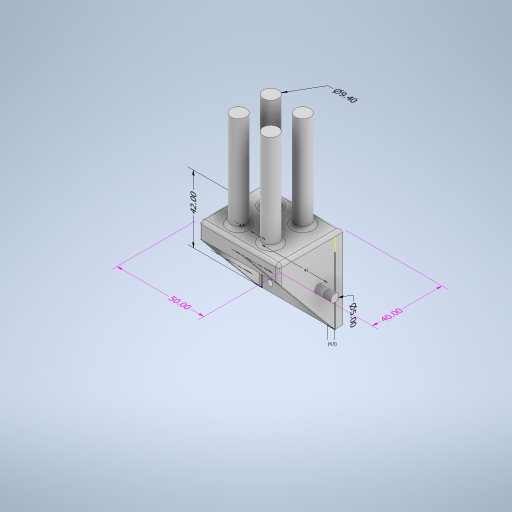
# Autodesk Inventor part: Attache moteur 3.0 renforcée
Saved by Autodesk Inventor 2023 (Build 270158000, 158)
## iProperties
Created: 2023-01-13
Part Number: Attache moteur 3.0 renforcée
Material: Générique
Document SubType Name: Modeling
Designer: pined
Density: 1 g/cm^3
Appearance: Par défaut
Mass: 44.8321 g
Surface Area: 196.652 cm^2
Volume: 44.8321 cm^3
Author: pined
Autodesk Inventor part; units mm, degrees
ref_plane "YZ Plane" through (0, 0, 0) normal (1, 0, 0) x (0, 1, 0)
ref_plane "XZ Plane" through (0, 0, 0) normal (0, 1, 0) x (-1, 0, 0)
ref_plane "XY Plane" through (0, 0, 0) normal (0, 0, 1) x (1, 0, 0)
sketch "Esquisse1" plane through (0, 0, 0) normal (1, 0, 0) x (0, 1, 0)
  line L0 (40.4154, 29.6476) -> (33.4154, 29.6476)
  line L1 (33.4154, 29.6476) -> (33.4154, -10.3524)
  line L2 (33.4154, -10.3524) -> (40.4154, -10.3524)
  line L3 (40.4154, -10.3524) -> (40.4154, 29.6476)
  line L4 (33.4154, -5.3524) -> (-16.5846, -5.3524)
  line L5 (-16.5846, -5.3524) -> (-16.5846, -10.3524)
  line L6 (-16.5846, -10.3524) -> (33.4154, -10.3524)
  line L7 (33.4154, -10.3524) -> (33.4154, -5.3524)
  point P0 (0, 0)
  point P1 (36.9154, -10.3524)
  point P2 (36.9154, 29.6476)
  point P3 (-16.5846, -7.8524)
  point P4 (33.4154, -7.8524)
  point P5 (33.4154, -10.3524)
  dimension "d0" = 40
  dimension "d1" = 7
  dimension "d2" = 5
  dimension "d3" = 50
  constraints: 16 end point, 4 midpoint, 4 parallel, 2 horizontal, 2 perpendicular, 1 point on line
  measures "d0" distance of point (36.915, -10.352) point (36.915, 29.648)
  measures "d1" distance between parallel lines of L1 L3
  measures "d2" distance between parallel lines of L6 L4
  measures "d3" distance of point (-16.585, -7.852) point (33.415, -7.852)
extrude "Extrusion1" add sketch "Esquisse1" along normal blind 50
sketch "Esquisse2" plane through (0, 33.4154, -5.3524) normal (0, -1, 0) x (1, 0, 0)
  line L0 (50, 35) -> (50, 0) projected
  line L1 (0, 0) -> (0, -5) projected
  line L2 (50, 35) -> (0, 0)
  line L3 (0, 0) -> (50, 0) projected
  line L4 (0, 35) -> (0, 0) projected
  line L5 (50, 0) -> (0, 35)
  line L6 (50, 3.0516) -> (4.3595, 35)
  line L7 (0, 35) -> (50, 35) projected
  line L8 (0, 31.9484) -> (46.6722, -0.7221)
  line L9 (50, 31.9484) -> (4.3595, 0)
  line L10 (45.6405, 35) -> (0, 3.0516)
  line L11 (50, 35) -> (0, 35)
  line L12 (0, 35) -> (0, 31.9484)
  line L13 (0, 31.9484) -> (50, 31.9484)
  line L14 (50, 31.9484) -> (50, 35)
  point P0 (0, 5.3524)
  point P1 (25, 20.5516)
  point P2 (8.719, 31.9484)
  point P3 (41.281, 31.9484)
  point P4 (20.6405, 17.5)
  point P5 (4.3595, 0)
  point P6 (25, 14.4484)
  point P7 (45.6405, 0)
  point P8 (29.3595, 17.5)
  dimension "d6" = 2.5
  dimension "d7" = 2.5
  dimension "d8" = 2.5
  dimension "d9" = 2.5
  constraints: 20 end point, 6 parallel, 6 point on line, 1 horizontal, 1 perpendicular
  measures "d6" distance between parallel lines of L5 L6
  measures "d7" distance between parallel lines of L8 L5
  measures "d8" distance between parallel lines of L9 L2
  measures "d9" distance between parallel lines of L10 L2
extrude "Extrusion2" add sketch "Esquisse2" along normal blind 3 contours L0 L13 L2 | L2 L13 L10 L7 | L9 L6 L2 L13 | L2 L6 L10 L13 | L10 L13 L6 L7 | L0 L5 L9 L6 | L9 L5 L2 L6 | L2 L5 L10 L6 | L6 L13 L5 L7 | L3 L8 L9 L5 | L9 L8 L2 L5 | L2 L8 L10 L5 | L10 L5 L13 L6 | L5 L13 L4 | L9 L3 L2 L8 | L2 L4 L10 L8 | L10 L8 L13 L5
sketch "Esquisse7" plane through (4.3595, 33.4154, -5.3524) normal (0, 0, 1) x (1, 0, 0)
  point P0 (-4.3595, -33.4154)
sketch "Esquisse8" plane through (4.3595, 33.4154, -5.3524) normal (0, -1, 0) x (1, 0, 0)
  line L0 (0, 0) -> (20.6405, 14.4484) projected
  line L1 (20.6405, 14.4484) -> (20.6405, 0)
  line L2 (0, 0) -> (41.281, 0) projected
  point P0 (-4.3595, 5.3524)
  constraints: 2 end point, 1 midpoint
sketch "Esquisse10" plane through (0, 40.4154, 29.6476) normal (0, 1, 0) x (1, 0, 0)
  circle A0 centre (35, 30) radius 4.7
  circle A1 centre (35, 10) radius 4.7
  circle A2 centre (15, 10) radius 4.7
  circle A3 centre (15, 30) radius 4.7
  line L0 (50, 40) -> (50, 0) projected
  line L1 (0, 40) -> (50, 40) projected
  point P0 (0, 29.6476)
  dimension "d40" = 20
  dimension "d41" = 20
  dimension "d42" = 20
  dimension "d43" = 20
  dimension "d44" = 9.4
  dimension "d45" = 9.4
  dimension "d46" = 9.4
  dimension "d47" = 9.4
  dimension "d48" = 15
  dimension "d49" = 15
  dimension "d50" = 10
  dimension "d51" = 10
  constraints: 4 centre point
  measures "d40" distance of A1.centre A0.centre
  measures "d41" distance of A3.centre A0.centre
  measures "d42" distance of A2.centre A3.centre
  measures "d43" distance of A2.centre A1.centre
  measures "d44" diameter of A0
  measures "d45" diameter of A1
  measures "d46" diameter of A3
  measures "d47" diameter of A2
  measures "d48" distance from line of A0.centre L0
  measures "d49" distance from line of A1.centre L0
  measures "d50" distance from line of A0.centre L1
  measures "d51" distance from line of A3.centre L1
extrude "Extrusion8" add sketch "Esquisse10" along normal blind 60
fillet "Congé1" radius 2 4 edges at (30.3, 40.4154, -0.3524) (30.3, 40.4154, 19.6476) (10.3, 40.4154, -0.3524) (10.3, 40.4154, 19.6476)
fillet "Congé2" radius 2 6 edges at (50, 40.4154, 9.6476) (25, 40.4154, -10.3524) (0, 40.4154, 9.6476) (0, 35.4154, 29.6476) (25, 40.4154, 29.6476) (50, 35.4154, 29.6476)
fillet "Congé5" radius 1.5 9 edges at (10.3203, 33.4154, 19.3718) (35.3203, 33.4154, 1.8718) (16.8595, 33.4154, 20.8976) (33.1405, 33.4154, 20.8976) (39.6797, 33.4154, 19.3718) (14.6797, 33.4154, 1.8718) (25, 33.4154, 26.5959) (10.3203, 33.4154, 4.9234) (39.6797, 33.4154, 4.9234)
fillet "Congé6" radius 1.5 1 edges at (25, 31.1654, 9.0959)
sketch "Esquisse12" plane through (0, -16.5846, -10.3524) normal (0, -1, 0) x (1, 0, 0)
  line L0 (0, 8.0516) -> (0, 5) projected
  line L1 (48, 2) -> (50, 0) projected
  line L2 (0, 5) -> (50, 5)
  line L3 (50, 5) -> (50, 0)
  line L4 (50, 0) -> (0, 0)
  line L5 (0, 0) -> (0, 5)
  point P0 (0, 10.3524)
  constraints: 8 end point, 2 parallel, 1 horizontal, 1 perpendicular
extrude "Extrusion10" cut sketch "Esquisse12" against normal blind 5
sketch "Esquisse13" plane through (45.6405, 30.4154, -5.3524) normal (0, 0, 1) x (1, 0, 0)
  line L0 (-45.6405, -42) -> (-45.6405, 8) projected
  line L1 (-25, 0) -> (-45.6405, 0) projected
  line L2 (-45.6405, -42) -> (-41.1405, -42)
  line L3 (-41.1405, -42) -> (-41.1405, 0)
  line L4 (-41.1405, 0) -> (-45.6405, 0)
  line L5 (-45.6405, 0) -> (-45.6405, -42)
  line L6 (-16.281, 0) -> (4.3595, 0) projected
  line L7 (4.3595, -42) -> (4.3595, 8) projected
  line L8 (-0.1405, 0) -> (4.3595, 0)
  line L9 (4.3595, 0) -> (4.3595, -42)
  line L10 (4.3595, -42) -> (-0.1405, -42)
  line L11 (-0.1405, -42) -> (-0.1405, 0)
  point P0 (-45.6405, -30.4154)
  dimension "d87" = 41
  dimension "d88" = 4.5
  dimension "d89" = 4.5
  constraints: 16 end point, 4 parallel, 2 horizontal, 2 perpendicular, 2 point on line
  measures "d87" distance between parallel lines of L11 L3
  measures "d88" distance between parallel lines of L0 L3
  measures "d89" distance between parallel lines of L7 L11
sketch "Esquisse14" plane through (0, 33.4154, -0.4698) normal (0, -1, 0) x (1, 0, 0)
  line L0 (2, 30.1174) -> (48, 30.1174) projected
  line L1 (0, -9.8826) -> (0, 28.1174) projected
  line L2 (3, 30.1174) -> (0, 30.1174)
  line L3 (0, 30.1174) -> (0, -4.9612)
  line L4 (0, -4.9612) -> (3, -4.9612)
  line L5 (3, -4.9612) -> (3, 30.1174)
  line L6 (50, -4.8826) -> (50, -1.831) projected
  line L7 (47, 30.1174) -> (50, 30.1174)
  line L8 (50, 30.1174) -> (50, -4.8826)
  line L9 (50, -4.8826) -> (47, -4.8826)
  line L10 (47, -4.8826) -> (47, 30.1174)
  point P0 (0, 0.4698)
  point P1 (50, -1.831)
  dimension "d90" = 3
  dimension "d91" = 3
  constraints: 16 end point, 4 parallel, 3 point on line, 2 horizontal, 2 perpendicular
  measures "d90" distance of L2.start L2.end
  measures "d91" distance of L7.start L7.end
extrude "Extrusion11" add sketch "Esquisse14" along normal up to surface (45 mm away)
sketch "Esquisse15" plane through (3, 33.4154, 22.665) normal (1, 0, 0) x (0, 0, -1)
  line L0 (28.0174, -45) -> (-6.9826, -3)
  point P0 (22.665, -33.4154)
  constraints: 2 end point
extrude "Extrusion12" cut sketch "Esquisse15" against normal blind 10 fills toward (10.479, -24.032) open curves L0
fillet "Congé7" radius 2 1 edges at (0, 31.9154, 29.6476)
sketch "Esquisse16" plane through (47, 33.4154, 1.6302) normal (-1, 0, 0) x (0, 0, 1)
  line L0 (28.0174, -3) -> (-6.9826, -45)
  point P0 (-1.6302, -33.4154)
  constraints: 2 end point
extrude "Extrusion13" cut sketch "Esquisse16" against normal blind 10 fills toward (10.5558, -24.032) open curves L0
fillet "Congé8" radius 2 1 edges at (50, 31.9154, 29.6476)
sketch "Esquisse18" plane through (6.9752, 33.4154, -5.3524) normal (0, 0, 1) x (1, 0, 0)
  circle A0 centre (18.0248, -24) radius 9
  line L0 (-3.9752, -45) -> (40.0248, -45) projected
  line L1 (-3.9752, -3) -> (-3.9752, -45) projected
  line L2 (40.0248, -45) -> (40.0248, -3) projected
  point P0 (-6.9752, -33.4154)
  dimension "d117" = 18
  dimension "d118" = 21
  dimension "d119" = 22
  dimension "d153" = 44
  constraints: 1 centre point
  measures "d117" diameter of A0
  measures "d118" distance from line of L0 A0.centre
  measures "d119" distance from line of L1 A0.centre
  measures "d153" distance between parallel lines of L2 L1
extrude "Extrusion15" cut sketch "Esquisse18" against normal blind 5
sketch "Esquisse19" plane through (6.9752, 33.4154, -5.3524) normal (0, 0, 1) x (1, 0, 0)
  circle A0 centre (33.5248, -9) radius 1.75
  circle A1 centre (33.5248, -40) radius 1.75
  circle A2 centre (2.5248, -40) radius 1.75
  circle A3 centre (2.5248, -9) radius 1.75
  line L0 (-3.9752, -3) -> (-3.9752, -45) projected
  line L1 (40.0248, -45) -> (40.0248, -3) projected
  line L2 (-3.9752, -45) -> (40.0248, -45) projected
  point P0 (-6.9752, -33.4154)
  dimension "d133" = 3.5
  dimension "d134" = 3.5
  dimension "d135" = 3.5
  dimension "d136" = 3.5
  dimension "d137" = 31
  dimension "d138" = 31
  dimension "d139" = 31
  dimension "d140" = 31
  dimension "d141" = 44
  dimension "d142" = 6.5
  dimension "d143" = 6.5
  dimension "d144" = 6.5
  dimension "d145" = 5
  constraints: 4 centre point
  measures "d133" diameter of A0
  measures "d134" diameter of A1
  measures "d135" diameter of A2
  measures "d136" diameter of A3
  measures "d137" distance of A1.centre A0.centre
  measures "d138" distance of A2.centre A3.centre
  measures "d139" distance of A2.centre A1.centre
  measures "d140" distance of A3.centre A0.centre
  measures "d141" distance between parallel lines of L0 L1
  measures "d142" distance from line of A1.centre L1
  measures "d143" distance from line of L0 A2.centre
  measures "d144" distance from line of A0.centre L1
  measures "d145" distance from line of L2 A1.centre
extrude "Extrusion16" cut sketch "Esquisse19" against normal through all
sketch "Esquisse20" plane through (50, 0, 0) normal (1, 0, 0) x (0, 0, -1)
  circle A0 centre (-4.6476, 15.4154) radius 2.5
  line L0 (-27.6476, 38.4154) -> (10.3524, 38.4154) projected
  line L1 (10.3524, -11.5846) -> (10.3524, 38.4154) projected
  point P0 (0, 0)
  dimension "d154" = 5
  dimension "d155" = 23
  dimension "d156" = 15
  constraints: 1 centre point
  measures "d154" diameter of A0
  measures "d155" distance from line of L0 A0.centre
  measures "d156" distance from line of L1 A0.centre
extrude "Extrusion17" add sketch "Esquisse20" along normal blind 10
sketch "Esquisse21" plane through (0, 0, 0) normal (-1, 0, 0) x (0, 0, 1)
  circle A0 centre (4.6476, 15.4154) radius 2.5 projected
  circle A1 centre (4.6476, 15.4154) radius 2.5
  point P0 (0, 0)
  constraints: 1 centre point, 1 coincident
extrude "Extrusion18" add sketch "Esquisse21" along normal blind 10
thread "Filetage1" size "M5x0.8" class "6g" standard "ANSI Metric M Profile" length 5
thread "Filetage2" size "M5x0.8" class "6g" standard "ANSI Metric M Profile" length 5 offset 5
